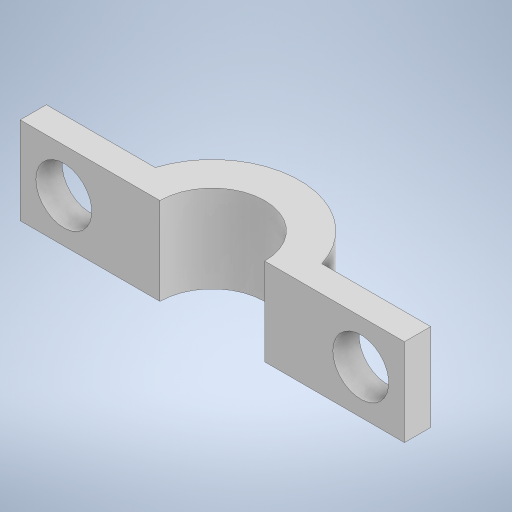
# Autodesk Inventor part: LazerHolder
Saved by Autodesk Inventor 2024 (Build 280153000, 153)
## iProperties
Created: 2025-05-07
Part Number: LazerHolder
Material: Generic
Document SubType Name: Modeling
Designer: Bjarni Heselmans
Density: 1 g/cm^3
Appearance: Default
Author: Bjarni Heselmans
Autodesk Inventor part; units mm, degrees
ref_plane "YZ Plane" through (0, 0, 0) normal (1, 0, 0) x (0, 1, 0)
ref_plane "XZ Plane" through (0, 0, 0) normal (0, 1, 0) x (-1, 0, 0)
ref_plane "XY Plane" through (0, 0, 0) normal (0, 0, 1) x (1, 0, 0)
sketch "Sketch1" plane through (0, 0, 0) normal (0, 0, 1) x (1, 0, 0)
  arc A0 (3, 0) -> (-3, 0) centre (0, 0) ccw
  line L0 (-3, 0) -> (-3, 1.5)
  line L1 (-4.7697, 1.5) -> (-11, 1.5)
  line L2 (-11, 1.5) -> (-11, 0)
  line L3 (0, -6.0366) -> (0, 6.6089)
  line L4 (3, 0) -> (3, 1.5)
  line L5 (4.7697, 1.5) -> (11, 1.5)
  line L6 (11, 1.5) -> (11, -1.5)
  arc A1 (4.7697, 1.5) -> (-4.7697, 1.5) centre (0, 0) ccw
  line L7 (3, 0) -> (15.1032, 0)
  line L8 (-11, 0) -> (-3, 0)
  line L9 (3, 0) -> (11, 0)
  dimension "d0" = 6
  dimension "d2" = 1.5
  dimension "d3" = 8
  dimension "d5" = 1.5
  dimension "d6" = 8
  constraints: 20 end point, 4 perpendicular, 4 point on circle, 3 vertical, 2 centre point, 2 coincident, 2 tangent, 1 horizontal, 1 midpoint, 1 point on line
  measures "d0" diameter of A0
  measures "d2" distance of L0.start L0.end
  measures "d3" distance of L0.end L1.end
  measures "d5" distance of L4.start L4.end
  measures "d6" distance of L4.end L5.end
extrude "Extrusion1" add sketch "Sketch1" along normal blind 5
sketch "Sketch2" plane through (-11, 1.5, 0) normal (0, 1, 0) x (1, 0, 0)
  line L0 (0, -5) -> (8, -5) projected
  line L1 (0, -5) -> (5, -5)
  line L2 (5, -5) -> (5, 0)
  line L3 (5, 0) -> (0, 0)
  line L4 (0, 0) -> (0, -5)
  circle A0 centre (2.5, -2.5) radius 1.6
  line L5 (11, 0) -> (11, -5)
  circle A1 centre (19.5, -2.5) radius 1.6
  dimension "d10" = 5
  dimension "d11" = 3.2
  constraints: 10 end point, 2 centre point, 2 parallel, 1 horizontal, 1 perpendicular, 1 symmetric about line, 1 vertical, 1 other
  measures "d10" distance of L3.end L2.end
  measures "d11" diameter of A0
extrude "Extrusion2" cut sketch "Sketch2" against normal blind 5 contours A0 | A1
body "Solid1"
